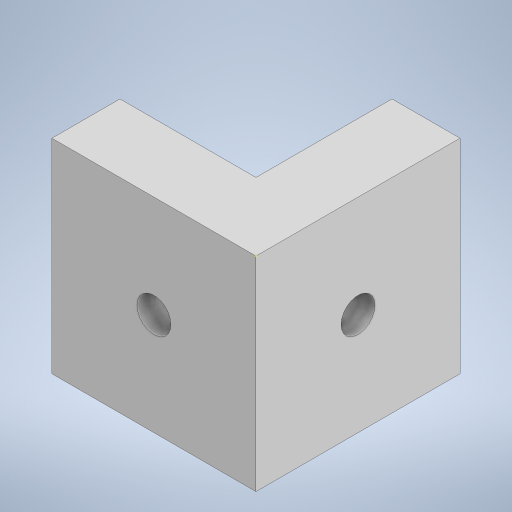
# Autodesk Inventor part: tunnel corner bracket_v02
Saved by Autodesk Inventor 2023 (Build 270158000, 158)
## iProperties
Created: 2021-04-13
Part Number: tunnel corner bracket_v02
Material: Generic
Document SubType Name: Modeling
Designer: KAMPFF-LAB-BEHAVIOR
Density: 1 g/cm^3
Appearance: Default
Author: KAMPFF-LAB-BEHAVIOR
Autodesk Inventor part; units mm, degrees
ref_plane "YZ Plane" through (0, 0, 0) normal (1, 0, 0) x (0, 1, 0)
ref_plane "XZ Plane" through (0, 0, 0) normal (0, 1, 0) x (-1, 0, 0)
ref_plane "XY Plane" through (0, 0, 0) normal (0, 0, 1) x (1, 0, 0)
sketch "Sketch34" plane through (0, 0, 0) normal (0, 0, 1) x (1, 0, 0)
  line L0 (0, 0) -> (30, 0)
  line L1 (30, 0) -> (30, -30)
  line L2 (30, -30) -> (0, -30)
  line L3 (0, -30) -> (0, 0)
  dimension "d112" = 30
  dimension "d113" = 30
  constraints: 8 end point, 2 parallel, 1 horizontal, 1 perpendicular
  measures "d112" distance of L1.end L2.end
  measures "d113" distance of L0.end L1.end
extrude "Extrusion25" add sketch "Sketch34" against normal blind 10
sketch "Sketch35" plane through (30, -30, 0) normal (1, 0, 0) x (0, 0, -1)
  line L0 (0, 30) -> (10, 30) projected
  line L1 (0, 30) -> (30, 30)
  line L2 (30, 30) -> (30, 0)
  line L3 (30, 0) -> (0, 0)
  line L4 (0, 0) -> (0, 30)
  dimension "d116" = 30
  dimension "d117" = 30
  constraints: 8 end point, 2 parallel, 1 horizontal, 1 perpendicular
  measures "d116" distance of L2.end L3.end
  measures "d117" distance of L1.end L2.end
extrude "Extrusion26" add sketch "Sketch35" against normal blind 10
sketch "Sketch36" plane through (0, 0, 0) normal (0, 0, 1) x (1, 0, 0)
  circle A0 centre (15, -15) radius 2.5
  point P0 (0, 0)
  dimension "d120" = 5
  constraints: 1 centre point
  measures "d120" diameter of A0
extrude "Extrusion27" cut sketch "Sketch36" against normal blind 10
sketch "Sketch37" plane through (30, -30, 0) normal (1, 0, 0) x (0, 0, -1)
  point P0 (0, 30)
sketch "Sketch38" plane through (30, -30, 0) normal (1, 0, 0) x (0, 0, -1)
  circle A0 centre (15, 15) radius 2.5
  point P0 (0, 30)
  dimension "d123" = 5
  constraints: 1 centre point
  measures "d123" diameter of A0
extrude "Extrusion28" cut sketch "Sketch38" against normal blind 10
sketch "Sketch39" plane through (30, -30, 0) normal (1, 0, 0) x (0, 0, -1)
  point P0 (0, 30)
sketch "Sketch42" plane through (0, 0, -10) normal (0, 0, -1) x (-1, 0, 0)
  circle A0 centre (-15, -15) radius 4
  point P0 (0, 0)
  dimension "d132" = 8
  constraints: 1 centre point
  measures "d132" diameter of A0
extrude "Extrusion31" cut sketch "Sketch42" against normal blind 5
sketch "Sketch43" plane through (20, -30, 0) normal (-1, 0, 0) x (0, 0, 1)
  circle A0 centre (-15, 15) radius 4
  point P0 (0, 30)
  dimension "d135" = 8
  constraints: 1 centre point
  measures "d135" diameter of A0
extrude "Extrusion32" cut sketch "Sketch43" against normal blind 5
body "Solid8"
